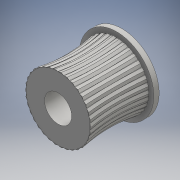
# Autodesk Inventor part: Roller2_v3
Saved by Autodesk Inventor 2016 (Build 200138000, 138)
## iProperties
Created: 2018-03-02
Part Number: Roller2_v3
Material: Generic
Document SubType Name: Modeling
Designer: Simon
Density: 1 g/cm^3
Appearance: Default
Author: Simon
Autodesk Inventor part; units mm, degrees
ref_plane "YZ Plane" through (0, 0, 0) normal (1, 0, 0) x (0, 1, 0)
ref_plane "XZ Plane" through (0, 0, 0) normal (0, 1, 0) x (-1, 0, 0)
ref_plane "XY Plane" through (0, 0, 0) normal (0, 0, 1) x (1, 0, 0)
sketch "Sketch1" plane through (0, 0, 0) normal (0, 0, 1) x (1, 0, 0)
  line L0 (0, 0) -> (0, 11)
  line L1 (0, 11) -> (-6, 11)
  line L2 (0, 0) -> (-6, 0)
  arc A0 (-6, 0) -> (-6, 11) centre (-36, 5.5) ccw
  line L3 (-6, 11) -> (-7, 11)
  line L4 (-7, 11) -> (-7, 12)
  line L5 (-7, 12) -> (0, 12)
  line L6 (0, 12) -> (0, 11)
  dimension "d1" = 11
  dimension "d2" = 6
  dimension "d3" = 6
  dimension "d4" = 5.5
  dimension "d5" = 1
  dimension "d6" = 1
  constraints: 14 end point, 4 perpendicular, 2 horizontal, 2 point on circle, 1 centre point, 1 vertical
  measures "d1" distance of L0.start L0.end
  measures "d2" distance of L0.end L1.end
  measures "d3" distance of L0.start L2.end
  measures "d4" distance edge to line of A0 L0
  measures "d5" distance of L1.end L3.end
  measures "d6" distance of L3.end L4.end
revolve "Revolution1" add sketch "Sketch1" angle 360 about axis through (0, 0, 0) along (0, 1, 0)
sketch "Sketch2" plane through (0, 12, 0) normal (0, 1, 0) x (1, 0, 0)
  line L0 (-1.95, 1.6432) -> (-1.95, -1.6432)
  arc A0 (-1.95, -1.6432) -> (-1.95, 1.6432) centre (0, 0) ccw
  arc A1 (-1.95, 1.6432) -> (-1.95, -1.6432) centre (0, 0) ccw
  constraints: 4 point on circle, 2 centre point, 2 end point, 1 coincident, 1 concentric
extrude "Extrusion1" cut sketch "Sketch2" against normal through all
sketch "Sketch3" plane through (0, 0, 0) normal (0, -1, 0) x (1, 0, 0)
  circle A0 centre (0, 0) radius 6 projected
  line L0 (5.9791, 0.5) -> (6.1611, 0)
  line L1 (5.9791, 0.5) -> (6.5112, 0.5) construction
  line L2 (6.1611, 0) -> (5.9791, -0.5)
  arc A1 (5.9791, -0.5) -> (5.9791, 0.5) centre (0, 0) ccw
  dimension "d13" = 1
  dimension "d14" = 70
  constraints: 6 end point, 4 point on circle, 1 centre point, 1 concentric, 1 equal length, 1 horizontal
  measures "d13" distance of L0.start L2.end
  measures "d14" angle of L0 L1
sketch "Sketch4" plane through (0, 0, 0) normal (0, 0, 1) x (1, 0, 0)
  arc A0 (6, 11) -> (6, 0) centre (36, 5.5) ccw projected
  point P0 (0, 0)
sweep "Sweep1" add profiles "Sketch3" path "Sketch4" contours A0 L0 L2
pattern_circular "Circular Pattern1" count 34 over 360 about axis through (0, -10, 0) along (0, 1, 0) of "Sweep1"
body "Solid1"
